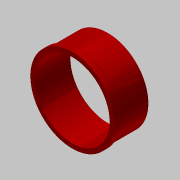
# Autodesk Inventor part: A1-19037-200-06 HCWI liner - pup - as cast
Saved by Autodesk Inventor 2017.3 (Build 213257000, 257)
## iProperties
Created: 2019-08-22
Part Number: A1-19037-200-06 HCWI liner - pup - as cast
Material: Iron, HCWI
Document SubType Name: Modeling
Designer: GVD
Density: 7.33517 g/cm^3
Appearance: Iron Gray(1)
Project: A1-19037--CNUL Albian CST laterals
Mass: 203382 g
Surface Area: 18277.3 cm^2
Volume: 27726.9 cm^3
Description: 28 1/2" ID x 1 1/4" WALL x 12 1/2" HCWI LINER, ASTM A532 CLASS III TYPE A, LEVEL 2, PF# 503368
Constructed By: Graeme_Van_Dongen
Project Name: CST laterals
Author: GVD
Autodesk Inventor part; units mm, degrees
ref_plane "YZ Plane" through (0, 0, 0) normal (1, 0, 0) x (0, 1, 0)
ref_plane "XZ Plane" through (0, 0, 0) normal (0, 1, 0) x (-1, 0, 0)
ref_plane "XY Plane" through (0, 0, 0) normal (0, 0, 1) x (1, 0, 0)
sketch "Sketch1" plane through (0, 0, 0) normal (0, 0, 1) x (1, 0, 0)
  circle A0 centre (0, 0) radius 361.95
  circle A1 centre (0, 0) radius 393.7
  dimension "d0" = 723.9
  dimension "d1" = 787.4
  constraints: 2 centre point, 2 coincident
  measures "d0" diameter of A0
  measures "d1" diameter of A1
extrude "Extrusion1" add sketch "Sketch1" along normal blind 304.8
sketch "Sketch2" plane through (0, 0, 304.8) normal (0, 0, 1) x (1, 0, 0)
  circle A0 centre (0, 0) radius 393.7 projected
  circle A1 centre (0, 0) radius 396.621
  circle A2 centre (0, 0) radius 399.796
  dimension "d4" = 793.242
  dimension "d5" = 799.592
  constraints: 2 centre point, 2 coincident
  measures "d4" diameter of A1
  measures "d5" diameter of A2
extrude "Extrusion2" add sketch "Sketch2" against normal blind 50.8 contours A1
extrude "Extrusion3" add sketch "Sketch2" against normal blind 25.4 contours A2
chamfer "Chamfer1" distance 2.921 angle 45 1 edges at (-393.7, 0, 254)
sketch "Sketch3" plane through (0, 0, 0) normal (0, 0, -1) x (-1, 0, 0)
  circle A0 centre (0, 0) radius 380.746
  circle A1 centre (0, 0) radius 361.95 projected
  dimension "d13" = 761.492
  constraints: 1 centre point, 1 coincident
  measures "d13" diameter of A0
extrude "Extrusion4" add sketch "Sketch3" along normal blind 12.7
fillet "Fillet1" radius 0.7937 2 edges at (380.746, 0, 0) (-396.621, 0, 279.4)
chamfer "Chamfer2" distance 0.7937 angle 45 1 edges at (380.746, 0, -12.7)
chamfer "Chamfer3" distance 0.7937 angle 45 1 edges at (-399.796, 0, 279.4)
sketch "Sketch4" plane through (0, 0, 0) normal (1, 0, 0) x (0, 1, 0)
  line L0 (396.621, 278.6062) -> (396.621, 254) construction
  line L1 (-399.796, 304.8) -> (399.796, 304.8) construction
  line L2 (396.621, 273.05) -> (394.8409, 271.2699)
  arc A0 (394.8409, 271.2699) -> (393.446, 267.9023) centre (398.2085, 267.9023) ccw
  line L3 (393.446, 267.9023) -> (393.446, 267.0852)
  arc A1 (393.446, 267.0852) -> (394.8409, 263.7176) centre (398.2085, 267.0852) ccw
  line L4 (394.8409, 263.7176) -> (396.621, 261.9375)
  line L5 (396.621, 261.9375) -> (396.621, 273.05)
  line L6 (0, -60.96) -> (0, 365.76) projected
  point P0 (0, 0)
  dimension "d23" = 11.1125
  dimension "d24" = 3.175
  dimension "d25" = 4.7625
  dimension "d26" = 31.75
  dimension "d27" = 45
  constraints: 8 end point, 4 point on circle, 4 tangent, 2 centre point, 2 point on line, 1 collinear, 1 equal radius, 1 perpendicular, 1 vertical
  measures "d23" distance of L2.start L4.end
  measures "d24" distance between parallel lines of L5 L3
  measures "d25" radius of A1
  measures "d26" distance from line of L1 L2.start
  measures "d27" angle of L5 L4
revolve "Revolution1" cut sketch "Sketch4" angle 360 about axis through (0, 0, -10) along (0, 0, 1)
sketch "Sketch7" plane through (0, 0, -12.7) normal (0, 0, -1) x (-1, 0, 0)
  circle A0 centre (0, 0) radius 361.95 projected
  circle A1 centre (0, 0) radius 393.7 projected
extrude "Extrusion7" add sketch "Sketch7" along normal mid plane 25.4
sketch "Sketch8" plane through (0, 0, 304.8) normal (0, 0, 1) x (1, 0, 0)
  circle A0 centre (0, 0) radius 399.796 projected
  circle A1 centre (0, 0) radius 361.95 projected
  circle A2 centre (0, 0) radius 406.146
  dimension "d43" = 6.35
  constraints: 1 centre point
  measures "d43" radial gap between concentric circles of A0 A2
extrude "Extrusion8" add sketch "Sketch8" along normal blind 12.7 and the other way blind 50.8 contours A0 | A2
chamfer "Chamfer4" distance 9.525 angle 45 1 edges at (-406.146, 0, 254)
equation "\"d10\" = -0.5 * d1 + 0.5 * d4"
body "Solid1"
